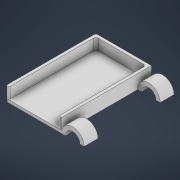
# Autodesk Inventor part: DripCatcher
Saved by Autodesk Inventor 2022 (Build 260153000, 153)
## iProperties
Created: 2024-03-01
Part Number: DripCatcher
Material: Všeobecné
Document SubType Name: Modeling
Designer: tada
Density: 1 g/cm^3
Appearance: Výchozí
Author: tada
Autodesk Inventor part; units mm, degrees
ref_plane "YZ Plane" through (0, 0, 0) normal (1, 0, 0) x (0, 1, 0)
ref_plane "XZ Plane" through (0, 0, 0) normal (0, 1, 0) x (-1, 0, 0)
ref_plane "XY Plane" through (0, 0, 0) normal (0, 0, 1) x (1, 0, 0)
sketch "Náčrt1" plane through (0, 0, 0) normal (0, 0, 1) x (1, 0, 0)
  circle A0 centre (0, 0) radius 5.25
  circle A1 centre (0, 0) radius 8.25
  line L0 (5.25, 0) -> (8.25, 0)
  line L1 (-8.25, 0) -> (-48.25, 0)
  line L2 (-8.25, 0) -> (-5.25, 0)
  line L3 (-48.25, 0) -> (-48.25, 2)
  line L4 (-48.25, 2) -> (-8.0039, 2)
  dimension "d0" = 10.5
  dimension "d1" = 3
  dimension "d2" = 40
  dimension "d3" = 2
  constraints: 10 end point, 5 point on circle, 3 horizontal, 2 centre point, 2 point on line, 1 coincident, 1 perpendicular, 1 vertical
  measures "d0" diameter of A0
  measures "d1" radial gap between concentric circles of A1 A0
  measures "d2" distance of L1.start L1.end
  measures "d3" distance between parallel lines of L4 L1
extrude "Vysunutí1" add sketch "Náčrt1" along normal blind 65 contours A0 L2 A1 L0 | L1 L3 L4 A1 picked at (7.1703, 0.6574)
sketch "Náčrt2" plane through (-48.25, 2, 0) normal (0, 1, 0) x (1, 0, 0)
  line L0 (40.2461, 0) -> (40.2461, -65) projected
  line L1 (56.5, 0) -> (56.5, -65) projected
  line L2 (40.2461, -10) -> (56.5, -10)
  line L3 (56.5, -10) -> (56.5, -55)
  line L4 (56.5, -55) -> (40.2461, -55)
  line L5 (40.2461, -55) -> (40.2461, -10)
  line L6 (40.2461, 0) -> (56.5, 0) projected
  line L7 (40.2461, -65) -> (56.5, -65) projected
  point P0 (48.25, 0)
  dimension "d6" = 10
  dimension "d7" = 10
  constraints: 8 end point, 2 parallel, 2 point on line, 1 horizontal, 1 perpendicular
  measures "d6" distance between parallel lines of L6 L2
  measures "d7" distance between parallel lines of L7 L4
extrude "Vysunutí2" cut sketch "Náčrt2" along normal mid plane 65 contours L2 L1 L4 L0
sketch "Náčrt3" plane through (-48.25, 2, 0) normal (0, 1, 0) x (1, 0, 0)
  line L0 (0, 0) -> (0, -65) projected
  line L1 (40.2461, 0) -> (0, 0) projected
  line L2 (0, 0) -> (40.2461, 0)
  line L3 (40.2461, -65) -> (56.5, -65) projected
  line L4 (40.2461, 0) -> (40.2461, -65)
  line L5 (40.2461, -65) -> (38.2461, -65)
  line L6 (38.2461, -65) -> (38.2461, -2)
  line L7 (38.2461, -2) -> (2, -2)
  line L8 (2, -2) -> (2, -65)
  line L9 (0, -65) -> (2, -65)
  line L10 (0, -65) -> (0, 0)
  point P0 (48.25, 0)
  dimension "d10" = 2
  dimension "d11" = 2
  dimension "d12" = 2
  dimension "d13" = 2
  dimension "d14" = 2
  constraints: 16 end point, 2 perpendicular, 1 collinear, 1 horizontal, 1 vertical
  measures "d10" distance of L3.start L5.end
  measures "d11" distance of L0.end L8.end
  measures "d12" distance between parallel lines of L7 L1
  measures "d13" distance between parallel lines of L4 L6
  measures "d14" distance between parallel lines of L0 L8
extrude "Vysunutí3" add sketch "Náčrt3" along normal blind 8
fillet "Zaoblení1" radius 2 2 edges at (-10.0039, 6, 2) (-46.25, 6, 2)
fillet "Zaoblení2" radius 1 2 edges at (-48.25, 5, 65) (-48.25, 5, 0)
fillet "Zaoblení3" radius 1 2 edges at (-46.25, 6, 65) (-10.0039, 6, 65)
